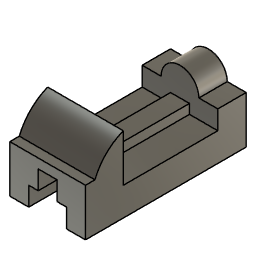
Robocon Task 1C 2 (Autodesk Fusion 360 design; units mm, degrees)
Autodesk Fusion 360 part; units mm, degrees
note: some values were not read from the file. Set by a fixed rule: which sketch regions a step uses.
sketch "Sketch1" plane through (0, 0, 0) normal (1, 0, 0) x (0, 1, 0)
  line L0 (0, 0) -> (17, 0)
  line L1 (17, 0) -> (17, 3)
  line L2 (17, 3) -> (0, 3)
  line L3 (0, 3) -> (0, 0)
  line L4 (0, 3) -> (4, 3)
  line L5 (4, 3) -> (4, 5)
  line L6 (4, 5) -> (0, 5)
  line L7 (0, 5) -> (0, 3)
  line L8 (4, 5) -> (4, 8)
  arc A0 (4, 8) -> (1, 5) centre (6, 3) ccw
  line L9 (1, 5) -> (1, 2.9999) construction
  line L10 (17, 3) -> (14, 3)
  line L11 (14, 3) -> (14, 5)
  line L12 (14, 5) -> (17, 5)
  line L13 (17, 5) -> (17, 3)
  dimension "d1" = 17
  dimension "d2" = 3
  dimension "d3" = 4
  dimension "d4" = 2
  dimension "d5" = 3
  dimension "d6" = 1
  dimension "d7" = 3
  dimension "d8" = 2
  constraint horizontal L0
  constraint vertical L1
  constraint horizontal L2
  constraint vertical L3
  constraint coincident L0.start L3.end
  constraint horizontal L4
  constraint vertical L5
  constraint horizontal L6
  constraint vertical L7
  constraint perpendicular L6 L8
  constraint vertical L9
  constraint coincident L6 A0.end
  constraint coincident L2 A0.centre
  constraint horizontal L10
  constraint vertical L11
  constraint horizontal L12
  constraint vertical L13
  measures "d1" distance of L0.start L0.end
  measures "d2" distance of L0.start L2.end
  measures "d3" distance of L2.end L4.end
  measures "d4" distance of L2.end L6.end
  measures "d5" distance of L5.end L8.end
  measures "d6" distance of L7 L9
  measures "d7" distance of L1.end L10.end
  measures "d8" distance of L1.end L12.end
extrude "Extrude1" add sketch "Sketch1" along normal blind 8 makes body 1
sketch "Sketch2" plane through (0, 14, 0) normal (0, -1, 0) x (1, 0, 0)
  line L0 (0, 5) -> (0, 3)
  line L1 (0, 3) -> (8, 3)
  line L2 (8, 3) -> (8, 5)
  line L3 (8, 5) -> (0, 5)
  circle A0 centre (4, 5) radius 2
  dimension "d11" = 4
  constraint midpoint L3 A0.centre
  measures "d11" diameter of A0
extrude "Extrude2" add sketch "Sketch2" against normal up to surface (3 mm away) contours L3 A0 picked at (4.1483, 5.65) bodies 1
sketch "Sketch3" plane through (0, 0, 0) normal (0, -1, 0) x (1, 0, 0)
  line L0 (0, 5) -> (0, 0)
  line L1 (0, 0) -> (8, 0)
  line L2 (8, 0) -> (8, 5)
  line L3 (8, 5) -> (0, 5)
  line L4 (4, 0) -> (6, 0)
  line L5 (6, 0) -> (6, 2)
  line L6 (6, 2) -> (4, 2)
  line L7 (4, 2) -> (4, 0)
  line L8 (4, 2) -> (5, 2)
  line L9 (5, 2) -> (5, 4)
  line L10 (5, 4) -> (4, 4)
  line L11 (4, 4) -> (4, 2)
  line L12 (3, 2) -> (3, 4)
  line L13 (3, 4) -> (4, 4)
  line L14 (4, 2) -> (3, 2)
  line L15 (2, 2) -> (4, 2)
  line L16 (2, 0) -> (2, 2)
  line L17 (4, 0) -> (2, 0)
  dimension "d14" = 2
  dimension "d15" = 2
  dimension "d16" = 1
  dimension "d17" = 2
  constraint horizontal L4
  constraint vertical L5
  constraint horizontal L6
  constraint vertical L7
  constraint midpoint L1 L4.start
  constraint horizontal L8
  constraint vertical L9
  constraint horizontal L10
  constraint vertical L11
  constraint symmetric L4.start L11 L7.end
  constraint symmetric L4.end L11 L16.start
  constraint symmetric L5.end L11 L15.start
  constraint symmetric L6.end L11 L7.start
  constraint symmetric L8.end L11 L12.start
  constraint symmetric L9.end L11 L12.end
  constraint symmetric L10.end L11 L13.end
  measures "d14" distance of L4.start L4.end
  measures "d15" distance of L4.start L6.end
  measures "d16" distance of L6.end L8.end
  measures "d17" distance of L6.end L10.end
extrude "Extrude3" cut sketch "Sketch3" against normal blind 18 contours L1 L7 L14 L15 L16 L17 | L1 L4 L5 L6 L7 L8 | L6 L8 L9 L10 L11 | L11 L12 L13 L14 L15 bodies 1
sketch "Sketch4" plane through (0, 14, 0) normal (0, -1, 0) x (1, 0, 0)
  line L0 (3, 3) -> (3, 4)
  line L1 (3, 4) -> (5, 4)
  line L2 (5, 4) -> (5, 3)
  line L3 (5, 3) -> (8, 3)
  line L4 (8, 3) -> (8, 5)
  line L5 (8, 5) -> (6, 5)
  arc A0 (6, 5) -> (2, 5) centre (4, 5) ccw
  line L6 (2, 5) -> (0, 5)
  line L7 (0, 5) -> (0, 3)
  line L8 (0, 3) -> (3, 3)
  line L9 (3, 3) -> (3, 4)
  line L10 (5, 4) -> (5, 3)
  line L11 (3, 4) -> (5, 4)
  constraint coincident L0.start L8.end
  constraint coincident L0.end L1.start
  constraint coincident L1.end L2.start
  constraint coincident L2.end L3.start
surface "Extrude4" add extruded along (0, -1, 0) between 0 and 10 path "Sketch4" along L9 L11 L10 separate body makes body 2
